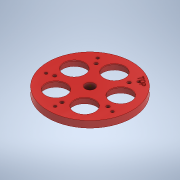
# Autodesk Inventor part: filterHolderBackPiece
Saved by Autodesk Inventor 2022.1 (Build 261234000, 234)
## iProperties
Created: 2020-04-12
Part Number: filterHolderBackPiece
Material: PBT Plastic
Document SubType Name: Modeling
Designer: robst
Density: 1.31 g/cm^3
Appearance: Orange-Red
wheelOuterDiameter: 4.501 in
wheelFilterDiameter: 2.611 in
filterThreadDiameter: 1.125 in
numberOfFilters: 5.000 ul
d5: 360.00 deg
distanceBetweenFilters: 0.500 in
distanceFromFilterToEdge: 0.375 in
wheelFilterCircumference: 8.200 in
filterDiameter: 1.140 in
Author: robst
Autodesk Inventor part; units mm, degrees
ref_plane "YZ Plane" through (0, 0, 0) normal (1, 0, 0) x (0, 1, 0)
ref_plane "XZ Plane" through (0, 0, 0) normal (0, 1, 0) x (-1, 0, 0)
ref_plane "XY Plane" through (0, 0, 0) normal (0, 0, 1) x (1, 0, 0)
sketch "Sketch1" plane through (0, 0, 0) normal (0, 1, 0) x (-1, 0, 0)
  circle A0 centre (0, 0) radius 57.1686
  circle A1 centre (0, 0) radius 33.1656 construction
  circle A2 centre (0, -33.1656) radius 14.2875
  circle A3 centre (31.5424, -10.2487) radius 14.2875
  circle A4 centre (19.4943, 26.8315) radius 14.2875
  circle A5 centre (-19.4943, 26.8315) radius 14.2875
  circle A6 centre (-31.5424, -10.2487) radius 14.2875
  dimension "wheelFilterDiameter" = 66.3312
  dimension "wheelOuterDiameter" = 114.3372
  dimension "filterThreadDiameter" = 28.575
  dimension "d5" = 360
  constraints: 6 centre point, 2 coincident, 1 vertical alignment, 13 other
  measures "wheelOuterDiameter" diameter of A0
  measures "filterThreadDiameter" diameter of A2
extrude "Extrusion5" add sketch "Sketch1" against normal blind 8.89
sketch "Sketch5" plane through (0, 0, 0) normal (0, 1, 0) x (1, 0, 0)
  arc A0 (35.921, 35.921) -> (0, 50.8) centre (0, 0) ccw construction
  line L0 (0, 0) -> (0, 50.8) construction
  line L1 (0, 0) -> (35.921, 35.921) construction
  line L2 (0, 0) -> (50.8, 0) construction
  line L3 (23.0912, 41.7997) -> (25.7305, 46.4819)
  line L4 (25.7305, 46.4819) -> (23.9488, 47.4861)
  line L5 (23.9488, 47.4861) -> (24.303, 48.1144)
  line L6 (24.303, 48.1144) -> (28.572, 45.7081)
  line L7 (28.572, 45.7081) -> (28.2178, 45.0798)
  line L8 (28.2178, 45.0798) -> (26.4362, 46.084)
  line L9 (26.4362, 46.084) -> (23.797, 41.4019)
  line L10 (23.797, 41.4019) -> (23.0912, 41.7997)
  spline S0 degree 2 poles (32.7583, 41.9026) (32.8009, 41.3717) (32.4178, 40.1854) (31.9717, 39.5691) knots 0 0 0 1 2 2 2
  spline S1 degree 2 poles (31.9717, 39.5691) (31.5371, 38.9689) (30.5291, 38.2167) (30.0034, 38.0971) knots 0 0 0 1 2 2 2
  spline S2 degree 2 poles (30.0034, 38.0971) (29.4502, 37.9731) (28.4083, 38.2273) (27.9242, 38.5778) knots 0 0 0 1 2 2 2
  spline S3 degree 2 poles (27.9242, 38.5778) (27.424, 38.9399) (26.8699, 39.8594) (26.8182, 40.403) knots 0 0 0 1 2 2 2
  spline S4 degree 2 poles (26.8182, 40.403) (26.7716, 40.9368) (27.1656, 42.1213) (27.606, 42.7295) knots 0 0 0 1 2 2 2
  spline S5 degree 2 poles (27.606, 42.7295) (28.055, 43.3498) (29.0467, 44.0711) (29.5771, 44.2055) knots 0 0 0 1 2 2 2
  spline S6 degree 2 poles (29.5771, 44.2055) (30.1027, 44.3251) (31.1533, 44.083) (31.6495, 43.7238) knots 0 0 0 1 2 2 2
  spline S7 degree 2 poles (31.6495, 43.7238) (32.1536, 43.3588) (32.707, 42.4215) (32.7583, 41.9026) knots 0 0 0 1 2 2 2
  spline S8 degree 2 poles (31.2874, 40.0645) (31.6408, 40.5527) (31.9762, 41.4625) (31.9637, 41.8496) knots 0 0 0 1 2 2 2
  spline S9 degree 2 poles (31.9637, 41.8496) (31.9531, 42.2477) (31.5862, 42.9035) (31.2421, 43.1527) knots 0 0 0 1 2 2 2
  spline S10 degree 2 poles (31.2421, 43.1527) (30.886, 43.4105) (30.1702, 43.5505) (29.7749, 43.4342) knots 0 0 0 1 2 2 2
  spline S11 degree 2 poles (29.7749, 43.4342) (29.3963, 43.324) (28.6378, 42.7144) (28.2902, 42.2342) knots 0 0 0 1 2 2 2
  spline S12 degree 2 poles (28.2902, 42.2342) (27.5863, 41.2618) (27.6552, 39.6385) (28.3395, 39.1431) knots 0 0 0 1 2 2 2
  spline S13 degree 2 poles (28.3395, 39.1431) (29.0238, 38.6477) (30.5835, 39.0921) (31.2874, 40.0645) knots 0 0 0 1 2 2 2
  spline S14 degree 2 poles (36.5539, 37.0614) (36.2883, 36.7688) (35.6016, 36.4313) (35.2491, 36.4177) knots 0 0 0 1 2 2 2
  spline S15 degree 2 poles (35.2491, 36.4177) (34.8058, 36.3997) (33.9572, 36.7363) (33.4743, 37.1746) knots 0 0 0 1 2 2 2
  line L11 (33.4743, 37.1746) -> (32.9659, 37.6361)
  line L12 (32.9659, 37.6361) -> (31.4386, 35.9534)
  line L13 (31.4386, 35.9534) -> (30.8387, 36.4979)
  line L14 (30.8387, 36.4979) -> (34.9357, 41.0119)
  line L15 (34.9357, 41.0119) -> (36.0697, 39.9826)
  spline S16 degree 2 poles (36.0697, 39.9826) (36.4721, 39.6174) (36.9159, 38.9744) (36.9956, 38.6286) knots 0 0 0 1 2 2 2
  spline S17 degree 2 poles (36.9956, 38.6286) (37.0919, 38.2276) (36.8958, 37.4382) (36.5539, 37.0614) knots 0 0 0 1 2 2 2
  spline S18 degree 2 poles (35.9117, 37.6109) (36.1242, 37.845) (36.2754, 38.3349) (36.2104, 38.594) knots 0 0 0 1 2 2 2
  spline S19 degree 2 poles (36.2104, 38.594) (36.154, 38.8186) (35.8433, 39.2407) (35.5617, 39.4964) knots 0 0 0 1 2 2 2
  line L16 (35.5617, 39.4964) -> (35.0642, 39.9479)
  line L17 (35.0642, 39.9479) -> (33.4307, 38.1482)
  line L18 (33.4307, 38.1482) -> (33.8404, 37.7764)
  spline S20 degree 2 poles (33.8404, 37.7764) (34.2062, 37.4443) (34.7623, 37.153) (35.0481, 37.1739) knots 0 0 0 1 2 2 2
  spline S21 degree 2 poles (35.0481, 37.1739) (35.3063, 37.1864) (35.7159, 37.395) (35.9117, 37.6109) knots 0 0 0 1 2 2 2
  dimension "d25" = 101.6
  dimension "d26" = 45
  constraints: 6 end point, 2 point on circle, 1 centre point, 1 coincident, 1 equal length, 1 horizontal, 1 vertical, 1 other
  measures "d25" diameter of A0
  measures "d26" angle of L2 L1
extrude "Extrusion6" cut sketch "Sketch5" against normal blind 1.016
sketch "Sketch6" plane through (0, -8.89, 0) normal (0, -1, 0) x (1, 0, 0)
  circle A0 centre (19.4943, 26.8315) radius 14.2875 projected
  circle A1 centre (19.4943, 26.8315) radius 16.1925
  point P0 (0, 0)
  dimension "d29" = 32.385
  constraints: 1 centre point, 1 coincident
  measures "d29" diameter of A1
extrude "Extrusion7" cut sketch "Sketch6" against normal blind 7.62 contours A0 | A1
pattern_circular "Circular Pattern2" count 5 over 360 about axis through (0, -10, 0) along (0, 1, 0) of "Extrusion7"
sketch "Sketch7" plane through (0, 0, 0) normal (0, 1, 0) x (1, 0, 0)
  circle A0 centre (0, 0) radius 6.477
  dimension "d35" = 12.954
  constraints: 1 centre point, 1 coincident
  measures "d35" diameter of A0
extrude "Extrusion8" cut sketch "Sketch7" against normal through all
sketch "Sketch8" plane through (0, 0, 0) normal (0, 1, 0) x (1, 0, 0)
  circle A0 centre (0, 0) radius 47.4531 construction
  circle A1 centre (19.4943, -26.8315) radius 14.2875 construction
  circle A2 centre (0, 0) radius 6.477 construction
  line L0 (0, 0) -> (27.8922, 38.3904) construction
  line L1 (0, 0) -> (0, 47.4531) construction
  circle A3 centre (0, 33.1656) radius 14.2875 construction
  point P0 (-27.8922, 38.3904)
  point P1 (-45.1306, -14.6638)
  point P2 (0, -47.4531)
  point P3 (45.1306, -14.6638)
  dimension "d38" = 36
  dimension "d41" = 360
  constraints: 4 end point, 2 coincident, 2 point on circle, 1 centre point, 1 tangent, 1 vertical alignment, 7 other
  measures "d38" angle of L0 L1
sketch "Sketch9" plane through (0, 0, 0) normal (0, 1, 0) x (1, 0, 0)
  line L0 (80.036, 0) -> (-80.036, 0) projected
  point P0 (27.8922, 38.3904)
  point P1 (-27.8922, 38.3904)
  point P2 (-45.1306, -14.6638)
  point P3 (0, -47.4531)
  point P4 (45.1306, -14.6638)
hole "Hole1" at (27.8922, 0, -38.3904) at (-27.8922, 0, -38.3904) at (-45.1306, 0, 14.6638) at (0, 0, 47.4531) at (45.1306, 0, 14.6638) direction (0, -1, 0) diameter 3.7973 end through all
sketch "Sketch10" plane through (0, -8.89, 0) normal (0, -1, 0) x (1, 0, 0)
  circle A0 centre (0, 0) radius 6.477 construction
  circle A1 centre (0, 0) radius 50.8 construction
  spline S0 degree 2 poles (-44.0461, 23.3584) (-43.705, 23.1938) (-43.3074, 22.6821) (-43.2405, 22.3847) knots 0 0 0 1 2 2 2
  spline S1 degree 2 poles (-43.2405, 22.3847) (-43.1655, 22.0286) (-43.2793, 21.3568) (-43.5047, 20.8896) knots 0 0 0 1 2 2 2
  line L0 (-43.5047, 20.8896) -> (-44.1379, 19.577)
  line L1 (-44.1379, 19.577) -> (-48.7134, 21.7841)
  line L2 (-48.7134, 21.7841) -> (-48.1285, 22.9966)
  spline S2 degree 2 poles (-48.1285, 22.9966) (-47.8924, 23.486) (-47.5933, 23.9451) (-47.3636, 24.1085) knots 0 0 0 1 2 2 2
  spline S3 degree 2 poles (-47.3636, 24.1085) (-47.114, 24.2943) (-46.5785, 24.3148) (-46.2893, 24.1753) knots 0 0 0 1 2 2 2
  spline S4 degree 2 poles (-46.2893, 24.1753) (-45.9667, 24.0197) (-45.6196, 23.4318) (-45.6198, 23.0617) knots 0 0 0 1 2 2 2
  line L3 (-45.6198, 23.0617) -> (-45.5976, 23.0509)
  spline S5 degree 2 poles (-45.5976, 23.0509) (-45.2896, 23.4052) (-44.4836, 23.5694) (-44.0461, 23.3584) knots 0 0 0 1 2 2 2
  spline S6 degree 2 poles (-44.326, 22.7118) (-44.5855, 22.837) (-44.9908, 22.8497) (-45.2168, 22.6844) knots 0 0 0 1 2 2 2
  spline S7 degree 2 poles (-45.2168, 22.6844) (-45.3607, 22.5756) (-45.5697, 22.2559) (-45.7217, 21.9408) knots 0 0 0 1 2 2 2
  line L4 (-45.7217, 21.9408) -> (-46.0544, 21.2511)
  line L5 (-46.0544, 21.2511) -> (-44.3636, 20.4355)
  line L6 (-44.3636, 20.4355) -> (-44.1258, 20.9287)
  spline S8 degree 2 poles (-44.1258, 20.9287) (-43.9326, 21.3291) (-43.785, 21.8246) (-43.8178, 22.0599) knots 0 0 0 1 2 2 2
  spline S9 degree 2 poles (-43.8178, 22.0599) (-43.8578, 22.2894) (-44.085, 22.5955) (-44.326, 22.7118) knots 0 0 0 1 2 2 2
  spline S10 degree 2 poles (-46.5098, 23.5001) (-46.673, 23.5788) (-46.9714, 23.5856) (-47.1008, 23.4973) knots 0 0 0 1 2 2 2
  spline S11 degree 2 poles (-47.1008, 23.4973) (-47.2539, 23.3883) (-47.4645, 23.0465) (-47.6201, 22.7239) knots 0 0 0 1 2 2 2
  line L7 (-47.6201, 22.7239) -> (-47.9009, 22.1418)
  line L8 (-47.9009, 22.1418) -> (-46.5624, 21.4961)
  line L9 (-46.5624, 21.4961) -> (-46.2297, 22.1858)
  spline S12 degree 2 poles (-46.2297, 22.1858) (-46.092, 22.4713) (-46.0208, 22.7706) (-46.0437, 22.9599) knots 0 0 0 1 2 2 2
  spline S13 degree 2 poles (-46.0437, 22.9599) (-46.0647, 23.1437) (-46.2948, 23.3964) (-46.5098, 23.5001) knots 0 0 0 1 2 2 2
  spline S14 degree 2 poles (-41.6038, 25.2552) (-41.5936, 25.1585) (-41.5492, 24.8272) (-41.5584, 24.6894) knots 0 0 0 1 2 2 2
  spline S15 degree 2 poles (-41.5584, 24.6894) (-41.5656, 24.498) (-41.6442, 24.1766) (-41.7899, 23.928) knots 0 0 0 1 2 2 2
  spline S16 degree 2 poles (-41.7899, 23.928) (-41.9085, 23.7255) (-42.2756, 23.4492) (-42.4953, 23.3919) knots 0 0 0 1 2 2 2
  spline S17 degree 2 poles (-42.4953, 23.3919) (-42.7073, 23.3395) (-43.1987, 23.4128) (-43.4189, 23.5419) knots 0 0 0 1 2 2 2
  spline S18 degree 2 poles (-43.4189, 23.5419) (-43.7599, 23.7417) (-44.0744, 24.3124) (-44.0297, 24.7061) knots 0 0 0 1 2 2 2
  spline S19 degree 2 poles (-44.0297, 24.7061) (-43.9953, 25.0581) (-43.6499, 25.8673) (-43.4188, 26.3187) knots 0 0 0 1 2 2 2
  line L10 (-43.4188, 26.3187) -> (-43.5253, 26.3812)
  spline S20 degree 2 poles (-43.5253, 26.3812) (-43.7171, 26.4936) (-44.0238, 26.5158) (-44.1537, 26.4488) knots 0 0 0 1 2 2 2
  spline S21 degree 2 poles (-44.1537, 26.4488) (-44.2836, 26.3818) (-44.5052, 26.1013) (-44.601, 25.9379) knots 0 0 0 1 2 2 2
  spline S22 degree 2 poles (-44.601, 25.9379) (-44.7134, 25.7461) (-44.9036, 25.161) (-44.9454, 24.8372) knots 0 0 0 1 2 2 2
  line L11 (-44.9454, 24.8372) -> (-44.9642, 24.8052)
  line L12 (-44.9642, 24.8052) -> (-45.5289, 25.1361)
  spline S23 degree 2 poles (-45.5289, 25.1361) (-45.482, 25.3138) (-45.2535, 25.9481) (-45.0891, 26.2287) knots 0 0 0 1 2 2 2
  spline S24 degree 2 poles (-45.0891, 26.2287) (-44.8892, 26.5697) (-44.51, 26.9725) (-44.2633, 27.076) knots 0 0 0 1 2 2 2
  spline S25 degree 2 poles (-44.2633, 27.076) (-44.0222, 27.1781) (-43.4883, 27.1038) (-43.1793, 26.9228) knots 0 0 0 1 2 2 2
  line L13 (-43.1793, 26.9228) -> (-40.931, 25.6053)
  line L14 (-40.931, 25.6053) -> (-41.2557, 25.0512)
  line L15 (-41.2557, 25.0512) -> (-41.6038, 25.2552)
  line L16 (-42.0655, 25.5257) -> (-42.9784, 26.0606)
  spline S26 degree 2 poles (-42.9784, 26.0606) (-43.0771, 25.8513) (-43.3685, 25.2157) (-43.422, 24.9942) knots 0 0 0 1 2 2 2
  spline S27 degree 2 poles (-43.422, 24.9942) (-43.4836, 24.7344) (-43.3716, 24.2823) (-43.1229, 24.1366) knots 0 0 0 1 2 2 2
  spline S28 degree 2 poles (-43.1229, 24.1366) (-42.8388, 23.9701) (-42.3638, 24.1212) (-42.1848, 24.4266) knots 0 0 0 1 2 2 2
  spline S29 degree 2 poles (-42.1848, 24.4266) (-42.0328, 24.6859) (-42.0068, 25.2432) (-42.0655, 25.5257) knots 0 0 0 1 2 2 2
  spline S30 degree 2 poles (-39.5121, 27.5613) (-39.7357, 27.2354) (-40.3063, 26.8331) (-40.6427, 26.7794) knots 0 0 0 1 2 2 2
  spline S31 degree 2 poles (-40.6427, 26.7794) (-40.9758, 26.7234) (-41.7403, 26.9335) (-42.1544, 27.2176) knots 0 0 0 1 2 2 2
  spline S32 degree 2 poles (-42.1544, 27.2176) (-42.5685, 27.5018) (-43.0213, 28.1371) (-43.0968, 28.4635) knots 0 0 0 1 2 2 2
  spline S33 degree 2 poles (-43.0968, 28.4635) (-43.1758, 28.7923) (-43.0167, 29.497) (-42.7978, 29.816) knots 0 0 0 1 2 2 2
  spline S34 degree 2 poles (-42.7978, 29.816) (-42.6208, 30.074) (-42.144, 30.4558) (-41.9209, 30.5773) knots 0 0 0 1 2 2 2
  line L17 (-41.9209, 30.5773) -> (-41.3269, 30.1697)
  line L18 (-41.3269, 30.1697) -> (-41.3478, 30.1391)
  spline S35 degree 2 poles (-41.3478, 30.1391) (-41.435, 30.114) (-41.6783, 30.0214) (-41.829, 29.94) knots 0 0 0 1 2 2 2
  spline S36 degree 2 poles (-41.829, 29.94) (-41.9601, 29.8653) (-42.25, 29.6248) (-42.3431, 29.4891) knots 0 0 0 1 2 2 2
  spline S37 degree 2 poles (-42.3431, 29.4891) (-42.625, 29.0783) (-42.3462, 28.1531) (-41.7794, 27.7641) knots 0 0 0 1 2 2 2
  spline S38 degree 2 poles (-41.7794, 27.7641) (-41.2261, 27.3844) (-40.2742, 27.4402) (-39.9807, 27.8679) knots 0 0 0 1 2 2 2
  spline S39 degree 2 poles (-39.9807, 27.8679) (-39.8037, 28.1258) (-39.6961, 28.741) (-39.7389, 29.035) knots 0 0 0 1 2 2 2
  line L19 (-39.7389, 29.035) -> (-39.718, 29.0656)
  line L20 (-39.718, 29.0656) -> (-39.124, 28.658)
  spline S40 degree 2 poles (-39.124, 28.658) (-39.1402, 28.5543) (-39.198, 28.2445) (-39.2395, 28.1331) knots 0 0 0 1 2 2 2
  spline S41 degree 2 poles (-39.2395, 28.1331) (-39.2919, 27.9694) (-39.3979, 27.7276) (-39.5121, 27.5613) knots 0 0 0 1 2 2 2
  line L21 (-36.6315, 31.4756) -> (-37.1561, 30.8145)
  line L22 (-37.1561, 30.8145) -> (-39.4778, 30.8492)
  line L23 (-39.4778, 30.8492) -> (-39.443, 30.4957)
  line L24 (-39.443, 30.4957) -> (-38.1951, 29.5053)
  line L25 (-38.1951, 29.5053) -> (-38.5943, 29.0023)
  line L26 (-38.5943, 29.0023) -> (-42.7508, 32.301)
  line L27 (-42.7508, 32.301) -> (-42.3516, 32.804)
  line L28 (-42.3516, 32.804) -> (-39.9202, 30.8744)
  line L29 (-39.9202, 30.8744) -> (-40.2444, 33.0553)
  line L30 (-40.2444, 33.0553) -> (-39.748, 33.6808)
  line L31 (-39.748, 33.6808) -> (-39.4725, 31.4651)
  line L32 (-39.4725, 31.4651) -> (-36.6315, 31.4756)
  dimension "d50" = 101.6
  constraints: 1 centre point, 1 coincident, 1 other
  measures "d50" diameter of A1
extrude "Extrusion9" cut sketch "Sketch10" against normal blind 1.27
sketch "Sketch12" plane through (0, -8.89, 0) normal (0, -1, 0) x (1, 0, 0)
  circle A0 centre (0, 0) radius 38.1 construction
  line L0 (0, 0) -> (-36.2353, 11.7735) construction
  circle A1 centre (-31.5424, -10.2487) radius 16.1925 construction
  circle A2 centre (-19.4943, 26.8315) radius 16.1925 construction
  line L1 (-36.2353, 11.7735) -> (-37.8114, 4.681) construction
  line L2 (-36.2353, 11.7735) -> (-33.3414, 18.4379) construction
  circle A3 centre (-19.4943, 26.8315) radius 16.1925 construction
  point P0 (-22.3946, -30.8235)
  point P1 (22.3946, -30.8235)
  point P2 (36.2353, 11.7735)
  point P3 (0, 38.1)
  dimension "d54" = 76.2
  dimension "d57" = 360
  constraints: 6 end point, 3 point on circle, 2 coincident, 1 centre point, 1 equal length, 10 other
  measures "d54" diameter of A0
hole "Hole2" at (-36.2353, -8.89, 11.7735) at (-22.3946, -8.89, -30.8235) at (22.3946, -8.89, -30.8235) at (36.2353, -8.89, 11.7735) at (0, -8.89, 38.1) direction (0, 1, 0) diameter 4.4958 end through all clearance for "Flat Head Machine Screw (82)" size "#8" standard "Ansi Unified Screw Threads"
equation "\"wheelFilterDiameter\" = 0.318471 * wheelFilterCircumference"
equation "\"wheelOuterDiameter\" = filterDiameter + wheelFilterDiameter + 2 * distanceFromFilterToEdge"
equation "\"d23\" = filterWheelThickness"
equation "\"d27\" = textDepth"
equation "\"d29\" = filterMaxDiameter"
equation "\"d30\" = filterDepth"
equation "\"d35\" = centerHoleDiameter"
equation "\"distanceBetweenFilters\" = 12.7"
equation "\"distanceFromFilterToEdge\" = 9.525"
equation "\"filterDiameter\" = 28.956"
equation "\"filterWheelThickness\" = 8.89"
equation "\"textDepth\" = 1.016"
equation "\"filterMaxDiameter\" = 32.385"
equation "\"filterDepth\" = 7.62"
equation "\"centerHoleDiameter\" = 12.954"
equation "\"wheelFilterCircumference\" = 208.28"
body "Solid3"
